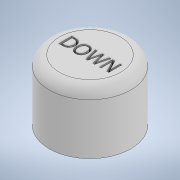
# Autodesk Inventor part: DOWN Button
Saved by Autodesk Inventor 2021 (Build 250183000, 183)
## iProperties
Created: 2021-03-30
Part Number: DOWN Button
Material: Generic
Document SubType Name: Modeling
Designer: eng1-177
Density: 1 g/cm^3
Appearance: Default
Author: eng1-177
Autodesk Inventor part; units mm, degrees
ref_plane "YZ Plane" through (0, 0, 0) normal (1, 0, 0) x (0, 1, 0)
ref_plane "XZ Plane" through (0, 0, 0) normal (0, 1, 0) x (-1, 0, 0)
ref_plane "XY Plane" through (0, 0, 0) normal (0, 0, 1) x (1, 0, 0)
sketch "Sketch1" plane through (0, 0, 0) normal (0, 1, 0) x (-1, 0, 0)
  circle A0 centre (0, 0) radius 10
  dimension "d0" = 20
  constraints: 1 centre point, 1 coincident
  measures "d0" diameter of A0
extrude "Extrusion1" add sketch "Sketch1" along normal blind 15
fillet "Fillet1" radius 2.5 1 edges at (10, 15, 0)
sketch "Sketch2" plane through (0, 15, 0) normal (0, 1, 0) x (1, 0, 0)
  line L0 (-6.4787, 1.7612) -> (2.2441, 1.7612) construction
  line L1 (2.2441, 1.7612) -> (2.2441, -4.757) construction
  line L2 (2.2441, -4.757) -> (-6.4787, -4.757) construction
  line L3 (-6.4787, -4.757) -> (-6.4787, 1.7612) construction
  spline S0 degree 2 poles (-3.658, 0.1068) (-3.658, -0.3273) (-4.01, -1.0261) (-4.3054, -1.2213) knots 0 0 0 1 2 2 2
  spline S1 degree 2 poles (-4.3054, -1.2213) (-4.5469, -1.3729) (-5.0427, -1.4756) (-5.428, -1.4756) knots 0 0 0 1 2 2 2
  line L4 (-5.428, -1.4756) -> (-6.1576, -1.4756)
  line L5 (-6.1576, -1.4756) -> (-6.1576, 1.6944)
  line L6 (-6.1576, 1.6944) -> (-5.4357, 1.6944)
  spline S2 degree 2 poles (-5.4357, 1.6944) (-4.9887, 1.6944) (-4.4801, 1.5608) (-4.3003, 1.4426) knots 0 0 0 1 2 2 2
  spline S3 degree 2 poles (-4.3003, 1.4426) (-3.9946, 1.2397) (-3.658, 0.5692) (-3.658, 0.1068) knots 0 0 0 1 2 2 2
  spline S4 degree 2 poles (-4.0973, 0.112) (-4.0973, 0.4767) (-4.3388, 0.9931) (-4.5777, 1.1395) knots 0 0 0 1 2 2 2
  spline S5 degree 2 poles (-4.5777, 1.1395) (-4.7472, 1.2397) (-5.13, 1.3296) (-5.4152, 1.3296) knots 0 0 0 1 2 2 2
  line L7 (-5.4152, 1.3296) -> (-5.7363, 1.3296)
  line L8 (-5.7363, 1.3296) -> (-5.7363, -1.1108)
  line L9 (-5.7363, -1.1108) -> (-5.4152, -1.1108)
  spline S6 degree 2 poles (-5.4152, -1.1108) (-5.1351, -1.1108) (-4.7113, -1.0209) (-4.5392, -0.9002) knots 0 0 0 1 2 2 2
  spline S7 degree 2 poles (-4.5392, -0.9002) (-4.3182, -0.7512) (-4.0973, -0.258) (-4.0973, 0.112) knots 0 0 0 1 2 2 2
  spline S8 degree 2 poles (-0.9581, 1.3322) (-0.7783, 1.1215) (-0.5779, 0.505) (-0.5779, 0.1094) knots 0 0 0 1 2 2 2
  spline S9 degree 2 poles (-0.5779, 0.1094) (-0.5779, -0.276) (-0.7732, -0.9002) (-0.9581, -1.1108) knots 0 0 0 1 2 2 2
  spline S10 degree 2 poles (-0.9581, -1.1108) (-1.1534, -1.3318) (-1.6697, -1.5424) (-1.9806, -1.5424) knots 0 0 0 1 2 2 2
  spline S11 degree 2 poles (-1.9806, -1.5424) (-2.3017, -1.5424) (-2.8154, -1.3241) (-3.003, -1.1108) knots 0 0 0 1 2 2 2
  spline S12 degree 2 poles (-3.003, -1.1108) (-3.1854, -0.9002) (-3.3806, -0.2811) (-3.3806, 0.1094) knots 0 0 0 1 2 2 2
  spline S13 degree 2 poles (-3.3806, 0.1094) (-3.3806, 0.5076) (-3.1828, 1.1138) (-3.0004, 1.3322) knots 0 0 0 1 2 2 2
  spline S14 degree 2 poles (-3.0004, 1.3322) (-2.8154, 1.5428) (-2.2991, 1.7612) (-1.9806, 1.7612) knots 0 0 0 1 2 2 2
  spline S15 degree 2 poles (-1.9806, 1.7612) (-1.6569, 1.7612) (-1.138, 1.5351) (-0.9581, 1.3322) knots 0 0 0 1 2 2 2
  spline S16 degree 2 poles (-1.0172, 0.1094) (-1.0172, 0.4228) (-1.1534, 0.9083) (-1.2767, 1.0676) knots 0 0 0 1 2 2 2
  spline S17 degree 2 poles (-1.2767, 1.0676) (-1.4026, 1.232) (-1.7571, 1.3964) (-1.978, 1.3964) knots 0 0 0 1 2 2 2
  spline S18 degree 2 poles (-1.978, 1.3964) (-2.2066, 1.3964) (-2.5508, 1.2371) (-2.6819, 1.0676) knots 0 0 0 1 2 2 2
  spline S19 degree 2 poles (-2.6819, 1.0676) (-2.8077, 0.9057) (-2.9413, 0.4176) (-2.9413, 0.1094) knots 0 0 0 1 2 2 2
  spline S20 degree 2 poles (-2.9413, 0.1094) (-2.9413, -0.5149) (-2.4173, -1.1776) (-1.978, -1.1776) knots 0 0 0 1 2 2 2
  spline S21 degree 2 poles (-1.978, -1.1776) (-1.5387, -1.1776) (-1.0172, -0.5149) (-1.0172, 0.1094) knots 0 0 0 1 2 2 2
  line L10 (3.4372, 1.6944) -> (2.6409, -1.4756)
  line L11 (2.6409, -1.4756) -> (2.1682, -1.4756)
  line L12 (2.1682, -1.4756) -> (1.5234, 1.1549)
  line L13 (1.5234, 1.1549) -> (0.8966, -1.4756)
  line L14 (0.8966, -1.4756) -> (0.4291, -1.4756)
  line L15 (0.4291, -1.4756) -> (-0.3801, 1.6944)
  line L16 (-0.3801, 1.6944) -> (0.054, 1.6944)
  line L17 (0.054, 1.6944) -> (0.6911, -0.9336)
  line L18 (0.6911, -0.9336) -> (1.323, 1.6944)
  line L19 (1.323, 1.6944) -> (1.752, 1.6944)
  line L20 (1.752, 1.6944) -> (2.3891, -0.9644)
  line L21 (2.3891, -0.9644) -> (3.0236, 1.6944)
  line L22 (3.0236, 1.6944) -> (3.4372, 1.6944)
  line L23 (6.0832, -1.4756) -> (5.6105, -1.4756)
  line L24 (5.6105, -1.4756) -> (4.2079, 1.2577)
  line L25 (4.2079, 1.2577) -> (4.2079, -1.4756)
  line L26 (4.2079, -1.4756) -> (3.8148, -1.4756)
  line L27 (3.8148, -1.4756) -> (3.8148, 1.6944)
  line L28 (3.8148, 1.6944) -> (4.4134, 1.6944)
  line L29 (4.4134, 1.6944) -> (5.6901, -0.8154)
  line L30 (5.6901, -0.8154) -> (5.6901, 1.6944)
  line L31 (5.6901, 1.6944) -> (6.0832, 1.6944)
  line L32 (6.0832, 1.6944) -> (6.0832, -1.4756)
  point P0 (0, 0)
  constraints: 2 other
extrude "Extrusion2" cut sketch "Sketch2" against normal blind 5
sketch "Sketch3" plane through (0, 0, 0) normal (0, -1, 0) x (1, 0, 0)
  circle A0 centre (0, 0) radius 7.5
  constraints: 1 centre point, 1 coincident
extrude "Extrusion3" cut sketch "Sketch3" against normal blind 2.5
body "Solid1"
